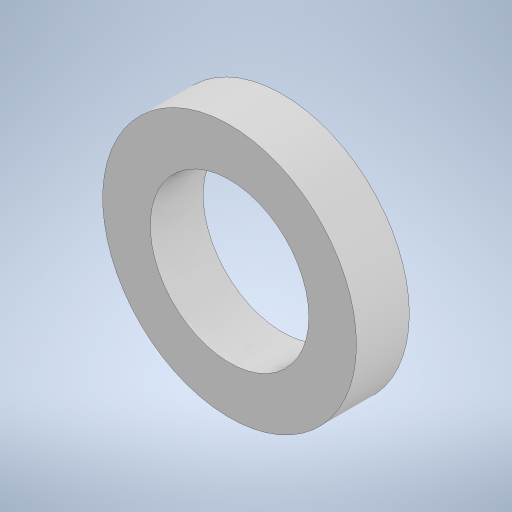
# Autodesk Inventor part: 15x24x5
Saved by Autodesk Inventor 2023 (Build 270158000, 158)
## iProperties
Created: 2023-01-17
Part Number: 15x24x5
Material: Generic
Document SubType Name: Modeling
Designer: caden
Density: 1 g/cm^3
Appearance: Default
Description: https://www.amazon.com/uxcell-6802-2RS-Bearing-1180802-Bearings/dp/B07FWGSFLN?crid=O2B8A4QKRUKF&keywords=Ball%2Bbearing%2B15x24x5&qid=1639878096&sprefix=ball%2Bbearing%2B15x24x5%2Caps%2C190&sr=8-5&th=1&linkCode=sl1&tag=howto045-20&linkId=8531902245b76ac8d0d906de28181aee&language=en_US&ref_=as_li_ss_tl
Author: caden
Autodesk Inventor part; units mm, degrees
ref_plane "YZ Plane" through (0, 0, 0) normal (1, 0, 0) x (0, 1, 0)
ref_plane "XZ Plane" through (0, 0, 0) normal (0, 1, 0) x (-1, 0, 0)
ref_plane "XY Plane" through (0, 0, 0) normal (0, 0, 1) x (1, 0, 0)
sketch "Sketch1" plane through (0, 0, 0) normal (0, 0, 1) x (1, 0, 0)
  circle A0 centre (0, 0) radius 12
  circle A1 centre (0, 0) radius 7.5
  dimension "d0" = 24
  dimension "d3" = 15
  constraints: 2 centre point, 2 coincident
  measures "d0" diameter of A0
  measures "d3" diameter of A1
extrude "Extrusion1" add sketch "Sketch1" along normal blind 5
body "Solid1"
